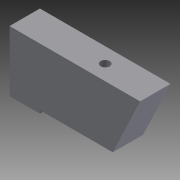
# Autodesk Inventor part: podpera_rameno
Saved by Autodesk Inventor 2015 (Build 190159000, 159)
## iProperties
Created: 2015-03-15
Part Number: podpera_rameno
Material: Generic
Document SubType Name: Modeling
Designer: Turboslimak
Density: 1 g/cm^3
Appearance: Default
Author: Turboslimak
Autodesk Inventor part; units mm, degrees
ref_plane "YZ Plane" through (0, 0, 0) normal (1, 0, 0) x (0, 1, 0)
ref_plane "XZ Plane" through (0, 0, 0) normal (0, 1, 0) x (-1, 0, 0)
ref_plane "XY Plane" through (0, 0, 0) normal (0, 0, 1) x (1, 0, 0)
sketch "Sketch1" plane through (0, 0, 0) normal (0, 1, 0) x (-1, 0, 0)
  line L0 (-21.5, 10) -> (21.5, 10)
  line L1 (21.5, 10) -> (21.5, -10)
  line L2 (21.5, -10) -> (11.5, -10)
  line L3 (11.5, -10) -> (11.5, -9)
  line L4 (11.5, -9) -> (-12.5, -9)
  line L5 (-12.5, -9) -> (-21.5, 10)
  line L6 (21.5, 10) -> (-21.5, 10)
  line L7 (21.5, 10) -> (21.5, -10)
  point P0 (0, 0)
  dimension "d0" = 43
  dimension "d2" = 10
  dimension "d3" = 1
  dimension "d4" = 24
  constraints: 16 end point, 1 horizontal, 1 parallel, 1 perpendicular
  measures "d0" distance of L0.start L0.end
  measures "d2" distance of L1.end L2.end
  measures "d3" distance of L2.end L3.end
  measures "d4" distance of L3.end L4.end
extrude "Extrusion1" add sketch "Sketch1" along normal blind 10
sketch "Sketch2" plane through (-21.5, 0, 10) normal (0, 0, 1) x (1, 0, 0)
  line L0 (0, 0) -> (0, 10) projected
  line L1 (0, 5) -> (26.5, 5)
  circle A0 centre (26.5, 5) radius 1.5
  point P0 (21.5, 0)
  dimension "d7" = 26.5
  dimension "d8" = 3
  constraints: 2 end point, 1 centre point, 1 coincident, 1 horizontal, 1 midpoint
  measures "d7" distance of L1.start L1.end
  measures "d8" diameter of A0
extrude "Extrusion2" cut sketch "Sketch2" against normal blind 19
body "Solid1"
